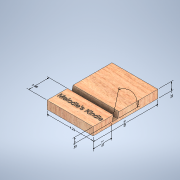
# Autodesk Inventor part: kindleStand
Saved by Autodesk Inventor 2020.2 (Build 242310000, 310)
## iProperties
Created: 2020-01-24
Part Number: kindleStand
Material: Wood (Birch)
Document SubType Name: Modeling
Designer: steele
Density: 0.55 g/cm^3
Appearance: Birch - Natural Polished
Author: steele
Autodesk Inventor part; units mm, degrees
ref_plane "YZ Plane" through (0, 0, 0) normal (1, 0, 0) x (0, 1, 0)
ref_plane "XZ Plane" through (0, 0, 0) normal (0, 1, 0) x (-1, 0, 0)
ref_plane "XY Plane" through (0, 0, 0) normal (0, 0, 1) x (1, 0, 0)
sketch "Sketch2" plane through (0, 0, 0) normal (0, 1, 0) x (-1, 0, 0)
  line L0 (53.975, 76.2) -> (-53.975, 76.2)
  line L1 (-53.975, 76.2) -> (-53.975, -76.2)
  line L2 (-53.975, -76.2) -> (53.975, -76.2)
  line L3 (53.975, -76.2) -> (53.975, 76.2)
  line L4 (53.975, 76.2) -> (-53.975, -76.2) construction
  line L5 (-53.975, 76.2) -> (53.975, -76.2) construction
  point P0 (0, 0)
  dimension "d0" = 107.95
  dimension "d1" = 152.4
  constraints: 12 end point, 2 midpoint, 2 parallel, 1 horizontal, 1 perpendicular
  measures "d0" distance of L0.start L0.end
  measures "d1" distance of L1.end L0.end
extrude "Extrusion1" add sketch "Sketch2" along normal blind 19.05
sketch "Sketch4" plane through (53.975, 0, 76.2) normal (1, 0, 0) x (0, 0, -1)
  line L0 (0, 19.05) -> (152.4, 19.05) projected
  line L1 (61.001, 19.05) -> (57.598, 6.35)
  line L2 (57.598, 6.35) -> (44.45, 6.35)
  line L3 (44.45, 6.35) -> (47.853, 19.05)
  line L4 (61.001, 19.05) -> (47.853, 19.05)
  line L5 (0, 0) -> (0, 19.05) projected
  point P0 (76.2, 0)
  point P1 (73.5162, 12.7)
  dimension "d27" = 12.7
  dimension "d28" = 44.45
  dimension "d29" = 75
  dimension "d46" = 12.7
  constraints: 8 end point, 2 parallel, 1 horizontal, 3 other
  measures "d28" distance from line of L5 L2.end
  measures "d29" angle of L3 L2
  measures "d46" distance between parallel lines of L1 L3
extrude "Extrusion3" cut sketch "Sketch4" against normal through all
sketch "Sketch6" plane through (0, 19.05, 0) normal (0, 1, 0) x (1, 0, 0)
  line L0 (-53.975, -28.347) -> (-53.975, -76.2) construction
  line L1 (-53.975, -50.8) -> (53.975, -50.8) construction
  line L2 (53.975, -76.2) -> (53.975, -28.347) construction
  line L3 (-53.975, -76.2) -> (53.975, -76.2) construction
  line L4 (-50.3934, -55.88) -> (-50.3934, -45.72)
  line L5 (-50.3934, -45.72) -> (-48.3723, -45.72)
  line L6 (-48.3723, -45.72) -> (-45.9639, -52.9141)
  spline S0 degree 2 poles (-45.9639, -52.9141) (-45.6309, -53.9208) (-45.4761, -54.4164) knots 0 0 0 1 1 1
  spline S1 degree 2 poles (-45.4761, -54.4164) (-45.3057, -53.8666) (-44.934, -52.7902) knots 0 0 0 1 1 1
  line L7 (-44.934, -52.7902) -> (-42.4947, -45.72)
  line L8 (-42.4947, -45.72) -> (-40.6903, -45.72)
  line L9 (-40.6903, -45.72) -> (-40.6903, -55.88)
  line L10 (-40.6903, -55.88) -> (-41.9836, -55.88)
  line L11 (-41.9836, -55.88) -> (-41.9836, -47.3772)
  line L12 (-41.9836, -47.3772) -> (-44.9495, -55.88)
  line L13 (-44.9495, -55.88) -> (-46.1575, -55.88)
  line L14 (-46.1575, -55.88) -> (-49.1002, -47.2301)
  line L15 (-49.1002, -47.2301) -> (-49.1002, -55.88)
  line L16 (-49.1002, -55.88) -> (-50.3934, -55.88)
  line L17 (-33.6511, -53.5026) -> (-32.3579, -53.6652)
  spline S2 degree 2 poles (-32.3579, -53.6652) (-32.6677, -54.7959) (-34.3171, -56.0426) (-35.5949, -56.0426) knots 0 0 0 1 2 2 2
  spline S3 degree 2 poles (-35.5949, -56.0426) (-37.2133, -56.0426) (-39.1028, -54.0524) (-39.1028, -52.2636) knots 0 0 0 1 2 2 2
  spline S4 degree 2 poles (-39.1028, -52.2636) (-39.1028, -50.4051) (-37.1901, -48.3529) (-35.6645, -48.3529) knots 0 0 0 1 2 2 2
  spline S5 degree 2 poles (-35.6645, -48.3529) (-34.1932, -48.3529) (-32.3192, -50.3663) (-32.3192, -52.1862) knots 0 0 0 1 2 2 2
  spline S6 degree 2 poles (-32.3192, -52.1862) (-32.3192, -52.2946) (-32.3269, -52.5191) knots 0 0 0 1 1 1
  line L18 (-32.3269, -52.5191) -> (-37.8174, -52.5191)
  spline S7 degree 2 poles (-37.8174, -52.5191) (-37.7477, -53.7349) (-36.5164, -55.0204) (-35.5949, -55.0204) knots 0 0 0 1 2 2 2
  spline S8 degree 2 poles (-35.5949, -55.0204) (-34.9056, -55.0204) (-33.9377, -54.2925) (-33.6511, -53.5026) knots 0 0 0 1 2 2 2
  line L19 (-37.7477, -51.497) -> (-33.6356, -51.497)
  spline S9 degree 2 poles (-33.6356, -51.497) (-33.7208, -50.5677) (-34.108, -50.0953) knots 0 0 0 1 1 1
  spline S10 degree 2 poles (-34.108, -50.0953) (-34.7043, -49.3751) (-35.6568, -49.3751) knots 0 0 0 1 1 1
  spline S11 degree 2 poles (-35.6568, -49.3751) (-36.5164, -49.3751) (-37.6857, -50.529) (-37.7477, -51.497) knots 0 0 0 1 2 2 2
  line L20 (-30.8246, -55.88) -> (-30.8246, -45.72)
  line L21 (-30.8246, -45.72) -> (-29.5778, -45.72)
  line L22 (-29.5778, -45.72) -> (-29.5778, -55.88)
  line L23 (-29.5778, -55.88) -> (-30.8246, -55.88)
  spline S12 degree 2 poles (-28.1065, -52.1939) (-28.1065, -50.1573) (-26.9681, -49.1738) knots 0 0 0 1 1 1
  spline S13 degree 2 poles (-26.9681, -49.1738) (-26.0234, -48.3529) (-24.6605, -48.3529) knots 0 0 0 1 1 1
  spline S14 degree 2 poles (-24.6605, -48.3529) (-23.1427, -48.3529) (-21.2144, -50.3431) (-21.2144, -52.0932) knots 0 0 0 1 2 2 2
  spline S15 degree 2 poles (-21.2144, -52.0932) (-21.2144, -53.5104) (-22.0663, -55.1443) (-23.6925, -56.0426) (-24.6605, -56.0426) knots 0 0 0 1 2 3 3 3
  spline S16 degree 2 poles (-24.6605, -56.0426) (-26.2015, -56.0426) (-28.1065, -54.0602) (-28.1065, -52.1939) knots 0 0 0 1 2 2 2
  spline S17 degree 2 poles (-26.821, -52.2016) (-26.821, -53.611) (-25.5897, -55.0204) (-24.6605, -55.0204) knots 0 0 0 1 2 2 2
  spline S18 degree 2 poles (-24.6605, -55.0204) (-23.7312, -55.0204) (-22.4999, -53.6033) (-22.4999, -52.1552) knots 0 0 0 1 2 2 2
  spline S19 degree 2 poles (-22.4999, -52.1552) (-22.4999, -50.7923) (-23.7389, -49.3829) (-24.6605, -49.3829) knots 0 0 0 1 2 2 2
  spline S20 degree 2 poles (-24.6605, -49.3829) (-25.5897, -49.3829) (-26.821, -50.7845) (-26.821, -52.2016) knots 0 0 0 1 2 2 2
  line L24 (-14.9728, -55.88) -> (-14.9728, -54.9507)
  spline S21 degree 2 poles (-14.9728, -54.9507) (-15.6698, -56.0426) (-17.0327, -56.0426) knots 0 0 0 1 1 1
  spline S22 degree 2 poles (-17.0327, -56.0426) (-17.9155, -56.0426) (-19.3869, -55.0746) (-20.2, -53.3323) (-20.2, -52.2016) knots 0 0 0 1 2 3 3 3
  spline S23 degree 2 poles (-20.2, -52.2016) (-20.2, -51.102) (-19.4643, -49.3054) (-18.0007, -48.3529) (-17.0947, -48.3529) knots 0 0 0 1 2 3 3 3
  spline S24 degree 2 poles (-17.0947, -48.3529) (-16.4287, -48.3529) (-15.391, -48.9105) (-15.0658, -49.3596) knots 0 0 0 1 2 2 2
  line L25 (-15.0658, -49.3596) -> (-15.0658, -45.72)
  line L26 (-15.0658, -45.72) -> (-13.819, -45.72)
  line L27 (-13.819, -45.72) -> (-13.819, -55.88)
  line L28 (-13.819, -55.88) -> (-14.9728, -55.88)
  spline S25 degree 2 poles (-18.9145, -52.2016) (-18.9145, -53.6188) (-17.7219, -55.0204) (-16.9088, -55.0204) knots 0 0 0 1 2 2 2
  spline S26 degree 2 poles (-16.9088, -55.0204) (-16.0957, -55.0204) (-14.9496, -53.6807) (-14.9496, -52.3101) knots 0 0 0 1 2 2 2
  spline S27 degree 2 poles (-14.9496, -52.3101) (-14.9496, -50.8) (-16.1112, -49.3829) (-16.963, -49.3829) knots 0 0 0 1 2 2 2
  spline S28 degree 2 poles (-16.963, -49.3829) (-17.7994, -49.3829) (-18.9145, -50.7458) (-18.9145, -52.2016) knots 0 0 0 1 2 2 2
  line L29 (-11.852, -55.88) -> (-11.852, -48.5155)
  line L30 (-11.852, -48.5155) -> (-10.6053, -48.5155)
  line L31 (-10.6053, -48.5155) -> (-10.6053, -55.88)
  line L32 (-10.6053, -55.88) -> (-11.852, -55.88)
  line L33 (-11.852, -47.1526) -> (-11.852, -45.72)
  line L34 (-11.852, -45.72) -> (-10.6053, -45.72)
  line L35 (-10.6053, -45.72) -> (-10.6053, -47.1526)
  line L36 (-10.6053, -47.1526) -> (-11.852, -47.1526)
  line L37 (-3.6745, -53.5026) -> (-2.3813, -53.6652)
  spline S29 degree 2 poles (-2.3813, -53.6652) (-2.691, -54.7959) (-4.3405, -56.0426) (-5.6182, -56.0426) knots 0 0 0 1 2 2 2
  spline S30 degree 2 poles (-5.6182, -56.0426) (-7.2367, -56.0426) (-9.1262, -54.0524) (-9.1262, -52.2636) knots 0 0 0 1 2 2 2
  spline S31 degree 2 poles (-9.1262, -52.2636) (-9.1262, -50.4051) (-7.2134, -48.3529) (-5.6879, -48.3529) knots 0 0 0 1 2 2 2
  spline S32 degree 2 poles (-5.6879, -48.3529) (-4.2166, -48.3529) (-2.3425, -50.3663) (-2.3425, -52.1862) knots 0 0 0 1 2 2 2
  spline S33 degree 2 poles (-2.3425, -52.1862) (-2.3425, -52.2946) (-2.3503, -52.5191) knots 0 0 0 1 1 1
  line L38 (-2.3503, -52.5191) -> (-7.8407, -52.5191)
  spline S34 degree 2 poles (-7.8407, -52.5191) (-7.771, -53.7349) (-6.5397, -55.0204) (-5.6182, -55.0204) knots 0 0 0 1 2 2 2
  spline S35 degree 2 poles (-5.6182, -55.0204) (-4.929, -55.0204) (-3.961, -54.2925) (-3.6745, -53.5026) knots 0 0 0 1 2 2 2
  line L39 (-7.771, -51.497) -> (-3.659, -51.497)
  spline S36 degree 2 poles (-3.659, -51.497) (-3.7442, -50.5677) (-4.1314, -50.0953) knots 0 0 0 1 1 1
  spline S37 degree 2 poles (-4.1314, -50.0953) (-4.7277, -49.3751) (-5.6802, -49.3751) knots 0 0 0 1 1 1
  spline S38 degree 2 poles (-5.6802, -49.3751) (-6.5397, -49.3751) (-7.7091, -50.529) (-7.771, -51.497) knots 0 0 0 1 2 2 2
  line L40 (-0.8092, -49.3209) -> (-1.1267, -47.4237)
  line L41 (-1.1267, -47.4237) -> (-1.1267, -45.72)
  line L42 (-1.1267, -45.72) -> (0.2904, -45.72)
  line L43 (0.2904, -45.72) -> (0.2904, -47.4237)
  line L44 (0.2904, -47.4237) -> (-0.0426, -49.3209)
  line L45 (-0.0426, -49.3209) -> (-0.8092, -49.3209)
  line L46 (1.39, -53.6807) -> (2.6213, -53.4871)
  spline S39 degree 2 poles (2.6213, -53.4871) (2.722, -54.2305) (3.6745, -55.0204) (4.5341, -55.0204) knots 0 0 0 1 2 2 2
  spline S40 degree 2 poles (4.5341, -55.0204) (5.3936, -55.0204) (6.23, -54.3157) (6.23, -53.8434) knots 0 0 0 1 2 2 2
  spline S41 degree 2 poles (6.23, -53.8434) (6.23, -53.4252) (5.8583, -53.1774) knots 0 0 0 1 1 1
  spline S42 degree 2 poles (5.8583, -53.1774) (5.6027, -53.0148) (4.5805, -52.7592) knots 0 0 0 1 1 1
  spline S43 degree 2 poles (4.5805, -52.7592) (3.2098, -52.4107) (2.1489, -51.9074) (1.5991, -51.0091) (1.5991, -50.4748) knots 0 0 0 1 2 3 3 3
  spline S44 degree 2 poles (1.5991, -50.4748) (1.5991, -49.9791) (2.0483, -49.1428) (2.4355, -48.864) knots 0 0 0 1 2 2 2
  spline S45 degree 2 poles (2.4355, -48.864) (2.7297, -48.6472) (3.7364, -48.3529) (4.3172, -48.3529) knots 0 0 0 1 2 2 2
  spline S46 degree 2 poles (4.3172, -48.3529) (5.1845, -48.3529) (6.4933, -48.8563) (7.1205, -49.7081) (7.2367, -50.4205) knots 0 0 0 1 2 3 3 3
  line L47 (7.2367, -50.4205) -> (6.0131, -50.5832)
  spline S47 degree 2 poles (6.0131, -50.5832) (5.928, -50.0101) (5.1303, -49.3751) (4.4024, -49.3751) knots 0 0 0 1 2 2 2
  spline S48 degree 2 poles (4.4024, -49.3751) (3.5428, -49.3751) (2.8072, -49.9482) (2.8072, -50.3276) knots 0 0 0 1 2 2 2
  spline S49 degree 2 poles (2.8072, -50.3276) (2.8072, -50.5677) (2.962, -50.7613) knots 0 0 0 1 1 1
  spline S50 degree 2 poles (2.962, -50.7613) (3.1092, -50.9626) (3.4422, -51.0943) knots 0 0 0 1 1 1
  spline S51 degree 2 poles (3.4422, -51.0943) (3.628, -51.164) (4.5418, -51.4195) knots 0 0 0 1 1 1
  spline S52 degree 2 poles (4.5418, -51.4195) (5.866, -51.768) (6.9192, -52.2171) (7.5155, -53.0767) (7.5155, -53.7195) knots 0 0 0 1 2 3 3 3
  spline S53 degree 2 poles (7.5155, -53.7195) (7.5155, -54.339) (6.7875, -55.4386) (5.4091, -56.0426) (4.5418, -56.0426) knots 0 0 0 1 2 3 3 3
  spline S54 degree 2 poles (4.5418, -56.0426) (3.1092, -56.0426) (1.5991, -54.8501) (1.39, -53.6807) knots 0 0 0 1 2 2 2
  line L48 (13.0369, -55.88) -> (13.0369, -45.72)
  line L49 (13.0369, -45.72) -> (14.3843, -45.72)
  line L50 (14.3843, -45.72) -> (14.3843, -50.7535)
  line L51 (14.3843, -50.7535) -> (19.4333, -45.72)
  line L52 (19.4333, -45.72) -> (21.2531, -45.72)
  line L53 (21.2531, -45.72) -> (16.994, -49.8398)
  line L54 (16.994, -49.8398) -> (21.439, -55.88)
  line L55 (21.439, -55.88) -> (19.6656, -55.88)
  line L56 (19.6656, -55.88) -> (16.0492, -50.7458)
  line L57 (16.0492, -50.7458) -> (14.3843, -52.3565)
  line L58 (14.3843, -52.3565) -> (14.3843, -55.88)
  line L59 (14.3843, -55.88) -> (13.0369, -55.88)
  line L60 (22.4147, -55.88) -> (22.4147, -48.5155)
  line L61 (22.4147, -48.5155) -> (23.6615, -48.5155)
  line L62 (23.6615, -48.5155) -> (23.6615, -55.88)
  line L63 (23.6615, -55.88) -> (22.4147, -55.88)
  line L64 (22.4147, -47.1526) -> (22.4147, -45.72)
  line L65 (22.4147, -45.72) -> (23.6615, -45.72)
  line L66 (23.6615, -45.72) -> (23.6615, -47.1526)
  line L67 (23.6615, -47.1526) -> (22.4147, -47.1526)
  line L68 (25.5588, -55.88) -> (25.5588, -48.5155)
  line L69 (25.5588, -48.5155) -> (26.6816, -48.5155)
  line L70 (26.6816, -48.5155) -> (26.6816, -49.561)
  spline S55 degree 2 poles (26.6816, -49.561) (27.4947, -48.3529) (29.0203, -48.3529) knots 0 0 0 1 1 1
  spline S56 degree 2 poles (29.0203, -48.3529) (29.6863, -48.3529) (30.8014, -48.833) (31.3589, -49.6074) (31.4673, -50.1418) knots 0 0 0 1 2 3 3 3
  spline S57 degree 2 poles (31.4673, -50.1418) (31.537, -50.4902) (31.537, -51.3576) knots 0 0 0 1 1 1
  line L71 (31.537, -51.3576) -> (31.537, -55.88)
  line L72 (31.537, -55.88) -> (30.2903, -55.88)
  line L73 (30.2903, -55.88) -> (30.2903, -51.404)
  spline S58 degree 2 poles (30.2903, -51.404) (30.2903, -50.6451) (29.996, -49.8862) (29.2603, -49.4371) (28.757, -49.4371) knots 0 0 0 1 2 3 3 3
  spline S59 degree 2 poles (28.757, -49.4371) (27.9594, -49.4371) (26.8055, -50.4515) (26.8055, -51.8609) knots 0 0 0 1 2 2 2
  line L74 (26.8055, -51.8609) -> (26.8055, -55.88)
  line L75 (26.8055, -55.88) -> (25.5588, -55.88)
  line L76 (38.2278, -55.88) -> (38.2278, -54.9507)
  spline S60 degree 2 poles (38.2278, -54.9507) (37.5308, -56.0426) (36.1679, -56.0426) knots 0 0 0 1 1 1
  spline S61 degree 2 poles (36.1679, -56.0426) (35.2851, -56.0426) (33.8138, -55.0746) (33.0006, -53.3323) (33.0006, -52.2016) knots 0 0 0 1 2 3 3 3
  spline S62 degree 2 poles (33.0006, -52.2016) (33.0006, -51.102) (33.7363, -49.3054) (35.1999, -48.3529) (36.1059, -48.3529) knots 0 0 0 1 2 3 3 3
  spline S63 degree 2 poles (36.1059, -48.3529) (36.7719, -48.3529) (37.8096, -48.9105) (38.1348, -49.3596) knots 0 0 0 1 2 2 2
  line L77 (38.1348, -49.3596) -> (38.1348, -45.72)
  line L78 (38.1348, -45.72) -> (39.3816, -45.72)
  line L79 (39.3816, -45.72) -> (39.3816, -55.88)
  line L80 (39.3816, -55.88) -> (38.2278, -55.88)
  spline S64 degree 2 poles (34.2861, -52.2016) (34.2861, -53.6188) (35.4787, -55.0204) (36.2918, -55.0204) knots 0 0 0 1 2 2 2
  spline S65 degree 2 poles (36.2918, -55.0204) (37.1049, -55.0204) (38.251, -53.6807) (38.251, -52.3101) knots 0 0 0 1 2 2 2
  spline S66 degree 2 poles (38.251, -52.3101) (38.251, -50.8) (37.0894, -49.3829) (36.2376, -49.3829) knots 0 0 0 1 2 2 2
  spline S67 degree 2 poles (36.2376, -49.3829) (35.4013, -49.3829) (34.2861, -50.7458) (34.2861, -52.2016) knots 0 0 0 1 2 2 2
  line L81 (41.3098, -55.88) -> (41.3098, -45.72)
  line L82 (41.3098, -45.72) -> (42.5566, -45.72)
  line L83 (42.5566, -45.72) -> (42.5566, -55.88)
  line L84 (42.5566, -55.88) -> (41.3098, -55.88)
  line L85 (49.5261, -53.5026) -> (50.8194, -53.6652)
  spline S68 degree 2 poles (50.8194, -53.6652) (50.5096, -54.7959) (48.8602, -56.0426) (47.5824, -56.0426) knots 0 0 0 1 2 2 2
  spline S69 degree 2 poles (47.5824, -56.0426) (45.9639, -56.0426) (44.0744, -54.0524) (44.0744, -52.2636) knots 0 0 0 1 2 2 2
  spline S70 degree 2 poles (44.0744, -52.2636) (44.0744, -50.4051) (45.9872, -48.3529) (47.5127, -48.3529) knots 0 0 0 1 2 2 2
  spline S71 degree 2 poles (47.5127, -48.3529) (48.9841, -48.3529) (50.8581, -50.3663) (50.8581, -52.1862) knots 0 0 0 1 2 2 2
  spline S72 degree 2 poles (50.8581, -52.1862) (50.8581, -52.2946) (50.8503, -52.5191) knots 0 0 0 1 1 1
  line L86 (50.8503, -52.5191) -> (45.3599, -52.5191)
  spline S73 degree 2 poles (45.3599, -52.5191) (45.4296, -53.7349) (46.6609, -55.0204) (47.5824, -55.0204) knots 0 0 0 1 2 2 2
  spline S74 degree 2 poles (47.5824, -55.0204) (48.2716, -55.0204) (49.2396, -54.2925) (49.5261, -53.5026) knots 0 0 0 1 2 2 2
  line L87 (45.4296, -51.497) -> (49.5416, -51.497)
  spline S75 degree 2 poles (49.5416, -51.497) (49.4564, -50.5677) (49.0692, -50.0953) knots 0 0 0 1 1 1
  spline S76 degree 2 poles (49.0692, -50.0953) (48.473, -49.3751) (47.5205, -49.3751) knots 0 0 0 1 1 1
  spline S77 degree 2 poles (47.5205, -49.3751) (46.6609, -49.3751) (45.4916, -50.529) (45.4296, -51.497) knots 0 0 0 1 2 2 2
  point P0 (0, 0)
  dimension "d50" = 25.4
  constraints: 2 end point, 2 horizontal, 2 point on line
  measures "d50" distance between parallel lines of L1 L3
extrude "Extrusion4" cut sketch "Sketch6" against normal blind 2.54
body "Solid1"
